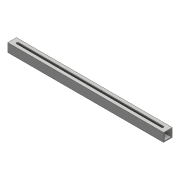
# Autodesk Inventor part: Rail
Saved by Autodesk Inventor 2016 (Build 200138000, 138)
## iProperties
Created: 2016-04-03
Part Number: Rail
Material: Generic
Document SubType Name: Modeling
Designer: Ariana
Density: 1 g/cm^3
Appearance: Default
Author: Ariana
Autodesk Inventor part; units mm, degrees
ref_plane "YZ Plane" through (0, 0, 0) normal (1, 0, 0) x (0, 1, 0)
ref_plane "XZ Plane" through (0, 0, 0) normal (0, 1, 0) x (-1, 0, 0)
ref_plane "XY Plane" through (0, 0, 0) normal (0, 0, 1) x (1, 0, 0)
sketch "Sketch1" plane through (0, 0, 0) normal (1, 0, 0) x (0, 1, 0)
  line L0 (0, 0) -> (25.4, 0)
  line L1 (25.4, 0) -> (25.4, 25.4)
  line L2 (25.4, 25.4) -> (0, 25.4)
  line L3 (0, 25.4) -> (0, 0)
  line L4 (22.86, 22.86) -> (22.86, 2.54)
  line L5 (22.86, 2.54) -> (2.54, 2.54)
  line L6 (2.54, 2.54) -> (2.54, 22.86)
  line L7 (2.54, 22.86) -> (22.86, 22.86)
  dimension "d0" = 2.54
  dimension "d1" = 25.4
  dimension "d2" = 25.4
  constraints: 16 end point, 4 parallel, 2 perpendicular, 1 horizontal, 3 other
  measures "d0" distance between parallel lines of L1 L4
  measures "d1" distance of L0.end L1.end
  measures "d2" distance of L0.start L0.end
extrude "Extrusion1" add sketch "Sketch1" along normal blind 457.2
sketch "Sketch2" plane through (0, 0, 25.4) normal (0, 0, 1) x (1, 0, 0)
  line L0 (15.875, 15.875) -> (441.325, 15.875)
  line L1 (444.5, 12.7) -> (444.5, 12.7)
  line L2 (441.325, 9.525) -> (15.875, 9.525)
  line L3 (12.7, 12.7) -> (12.7, 12.7)
  line L4 (457.2, 25.4) -> (457.2, 0) projected
  line L5 (0, 25.4) -> (0, 0) projected
  line L6 (0, 25.4) -> (457.2, 25.4) projected
  arc A0 (15.875, 15.875) -> (12.7, 12.7) centre (15.875, 12.7) ccw
  arc A1 (12.7, 12.7) -> (15.875, 9.525) centre (15.875, 12.7) ccw
  arc A2 (444.5, 12.7) -> (441.325, 15.875) centre (441.325, 12.7) ccw
  arc A3 (441.325, 9.525) -> (444.5, 12.7) centre (441.325, 12.7) ccw
  point P0 (12.7, 15.875)
  point P1 (12.7, 9.525)
  dimension "d5" = 6.35
  dimension "d6" = 12.7
  dimension "d7" = 12.7
  dimension "d8" = 9.525
  dimension "d9" = 3.175
  constraints: 8 end point, 8 point on circle, 8 tangent, 4 centre point, 4 point on line, 3 equal radius, 2 parallel, 1 horizontal, 1 perpendicular
  measures "d5" distance of point (12.7, 9.525) point (12.7, 15.875)
  measures "d6" distance between parallel lines of L4 L1
  measures "d7" distance between parallel lines of L5 L3
  measures "d8" distance between parallel lines of L6 L0
  measures "d9" radius of A0
extrude "Extrusion2" cut sketch "Sketch2" against normal blind 457.2
body "Solid1"
